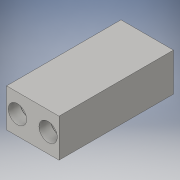
# Autodesk Inventor part: Part1
Saved by Autodesk Inventor 2016 (Build 200138000, 138)
## iProperties
Created: 2016-12-19
Part Number: Part1
Material: Generic
Document SubType Name: Modeling
Designer: Student
Density: 1 g/cm^3
Appearance: Default
Author: Student
Autodesk Inventor part; units mm, degrees
ref_plane "YZ Plane" through (0, 0, 0) normal (1, 0, 0) x (0, 1, 0)
ref_plane "XZ Plane" through (0, 0, 0) normal (0, 1, 0) x (-1, 0, 0)
ref_plane "XY Plane" through (0, 0, 0) normal (0, 0, 1) x (1, 0, 0)
sketch "Sketch1" plane through (0, 0, 0) normal (0, 0, 1) x (1, 0, 0)
  line L0 (-13.97, 10.16) -> (0, 10.16)
  line L1 (0, 10.16) -> (0, 0)
  line L2 (0, 0) -> (-13.97, 0)
  line L3 (-13.97, 0) -> (-13.97, 10.16)
  dimension "d0" = 13.97
  dimension "d1" = 10.16
  constraints: 8 end point, 2 parallel, 1 coincident, 1 horizontal, 1 perpendicular
  measures "d0" distance of L1.end L2.end
  measures "d1" distance of L0.end L1.end
extrude "Extrusion1" add sketch "Sketch1" along normal blind 30.48
sketch "Sketch2" plane through (0, 0, 0) normal (0, 0, -1) x (-1, 0, 0)
  line L0 (13.97, 10.16) -> (0, 10.16) projected
  line L1 (0, 10.16) -> (0, 0) projected
  line L2 (0, 0) -> (13.97, 0) projected
  line L3 (13.97, 0) -> (13.97, 10.16) projected
  circle A0 centre (2.8956, 5.08) radius 2.8194
  circle A1 centre (11.0744, 5.08) radius 2.8194
  dimension "d4" = 5.6388
  dimension "d5" = 5.6388
  dimension "d6" = 2.54
  dimension "d7" = 5.08
  dimension "d8" = 2.8956
  dimension "d9" = 2.8956
  constraints: 2 centre point
  measures "d4" diameter of A0
  measures "d5" diameter of A1
  measures "d7" distance from line of L0 A0.centre
  measures "d8" distance from line of L1 A0.centre
  measures "d9" distance from line of L3 A1.centre
extrude "Extrusion2" cut sketch "Sketch2" against normal blind 27.178 contours A0 | A1
sketch "Sketch3" plane through (0, 0, 0) normal (0, 0, -1) x (-1, 0, 0)
  circle A0 centre (2.8956, 5.08) radius 2.8194 projected
  circle A1 centre (11.0744, 5.08) radius 2.8194 projected
  circle A2 centre (2.8956, 5.08) radius 2.4447
  circle A3 centre (11.0744, 5.08) radius 2.4447
  point P0 (0, 0)
  dimension "d12" = 4.8895
  dimension "d13" = 4.8895
  constraints: 2 centre point, 2 coincident
  measures "d12" diameter of A2
  measures "d13" diameter of A3
extrude "Extrusion3" cut sketch "Sketch3" against normal blind 33.02 contours A2 | A3
chamfer "Chamfer1" distance 0.2032 angle 45 2 edges at (-0.4509, 5.08, 27.178) (-8.6297, 5.08, 27.178)
body "Solid1"
